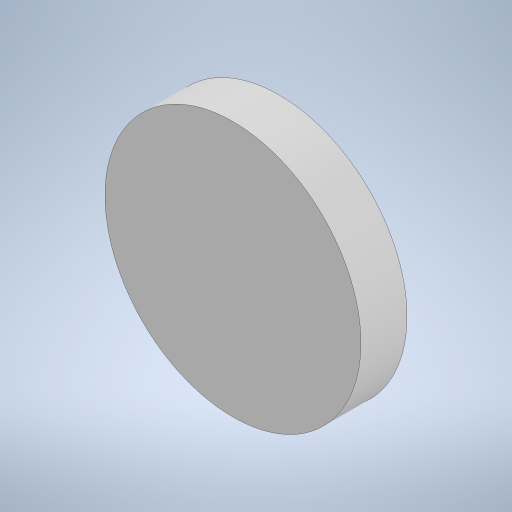
# Autodesk Inventor part: crucible_support
Saved by Autodesk Inventor 2023 (Build 270158000, 158)
## iProperties
Created: 2023-01-25
Part Number: crucible_support
Material: Generic
Document SubType Name: Modeling
Designer: remidm
Density: 1 g/cm^3
Appearance: Default
SupportHeight: 0.394 in
Author: remidm
Autodesk Inventor part; units mm, degrees
ref_plane "YZ Plane" through (0, 0, 0) normal (1, 0, 0) x (0, 1, 0)
ref_plane "XZ Plane" through (0, 0, 0) normal (0, 1, 0) x (-1, 0, 0)
ref_plane "XY Plane" through (0, 0, 0) normal (0, 0, 1) x (1, 0, 0)
sketch "Sketch1" plane through (0, 0, 0) normal (0, 0, 1) x (1, 0, 0)
  circle A0 centre (0, 0) radius 27.7794
  line L0 (-15.1761, -27.7794) -> (15.5731, -27.7794)
  circle A1 centre (0, 0) radius 26.4642
  dimension "d13" = 55.5588
  dimension "SupportThickness" = 1.3152
  constraints: 2 centre point, 2 coincident, 2 end point, 1 horizontal, 1 tangent
  measures "d13" diameter of A0
  measures "SupportThickness" radial gap between concentric circles of A0 A1
extrude "Extrusion1" add sketch "Sketch1" along normal blind 1.3152 contours A0 | A1
extrude "Extrusion3" add sketch "Sketch1" against normal blind 8.6848
equation "\"d13\" = 1.1 * CrucibleOuterDiameter"
equation "\"d1\" = SupportThickness"
equation "\"d15\" = SupportHeight - SupportThickness"
equation "\"CrucibleOuterDiameter\" = 50.508"
equation "\"SupportHeight\" = 10"
body "Solid1"
